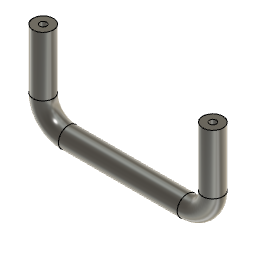
EWI_HANDLE v1 (Autodesk Fusion 360 design; units mm, degrees)
Autodesk Fusion 360 part; units mm, degrees
sketch "Sketch1" plane through (0, 0, 0) normal (0, 0, 1) x (1, 0, 0)
sketch "Sketch2" plane through (0, 0, 0) normal (0, 0, 1) x (1, 0, 0)
  circle A0 centre (0, 0) radius 3
  dimension "d1" = 6
  constraint coincident A0.centre origin
  measures "d1" diameter of A0
sketch "Sketch3" plane through (0, 0, 0) normal (0, 1, 0) x (1, 0, 0)
  line L0 (0, 0) -> (0, 17.5)
  line L1 (-7.5, 25) -> (-42.5, 25)
  line L2 (-50, 17.5) -> (-50, 0)
  arc A0 (0, 17.5) -> (-7.5, 25) centre (-7.5, 17.5) ccw
  arc A1 (-42.5, 25) -> (-50, 17.5) centre (-42.5, 17.5) ccw
  point P0 (0, 25)
  point P1 (-50, 25)
  dimension "d2" = 25
  dimension "d4" = 7.5
  dimension "d5" = 7.5
  constraint coincident L0.start origin
  constraint vertical L0
  constraint perpendicular L0 L1
  constraint perpendicular L1 L2
  constraint coincident P0 L0
  constraint coincident P0 L1
  constraint tangent L0 A0
  constraint tangent L1 A0
  constraint coincident P1 L1
  constraint coincident P1 L2
  constraint tangent L1 A1
  constraint tangent L2 A1
  measures "d2" distance of L0.start P0
  measures "d4" radius of A0
  measures "d5" radius of A1
sweep "Sweep1" add profiles "Sketch2" path "Sketch3" along L0 A0 L1 A1 L2 section 1
sketch "Sketch4" plane through (0, 0, 0) normal (0, 0, 1) x (1, 0, 0)
  circle A0 centre (0, 0) radius 1
  dimension "d12" = 2
  constraint coincident A0.centre origin
  measures "d12" diameter of A0
extrude "Extrude1" cut sketch "Sketch4" against normal blind 15
sketch "Sketch5" plane through (0, 0, 0) normal (0, 0, 1) x (-1, 0, 0)
  circle A0 centre (50, 0) radius 3
  circle A1 centre (50, 0) radius 1
  dimension "d15" = 2
  constraint concentric A0 A1
  measures "d15" diameter of A1
extrude "Extrude2" cut sketch "Sketch5" against normal blind 15 contours A1
